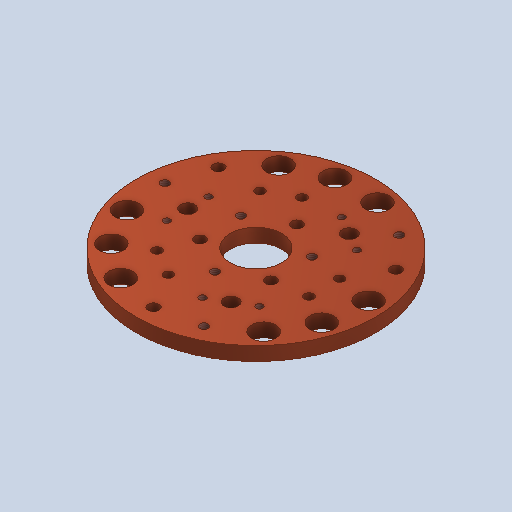
# Autodesk Inventor part: torsosc-frame-plate-v3
Saved by Autodesk Inventor 2026 (Build 300175050, 175E)
## iProperties
Created: 2018-11-20
Part Number: torsosc-frame-plate-v3
Material: Copper
Document SubType Name: Modeling
Designer: schanen
Density: 8.94 g/cm^3
Appearance: Copper - Satin
Mass: 121.653 g
Surface Area: 89.8116 cm^2
Volume: 13.6077 cm^3
Author: schanen
Autodesk Inventor part; units mm, degrees
ref_plane "YZ Plane" through (0, 0, 0) normal (1, 0, 0) x (0, 1, 0)
ref_plane "XZ Plane" through (0, 0, 0) normal (0, 1, 0) x (-1, 0, 0)
ref_plane "XY Plane" through (0, 0, 0) normal (0, 0, 1) x (1, 0, 0)
sketch "Sketch1" plane through (0, 0, 0) normal (0, 1, 0) x (-1, 0, 0)
  circle A0 centre (0, 0) radius 35
  circle A1 centre (0, 0) radius 7.5
  dimension "d0" = 70
  dimension "d129" = 15
  constraints: 2 centre point, 2 coincident
  measures "d0" diameter of A0
  measures "d129" diameter of A1
extrude "Extrusion1" add sketch "Sketch1" along normal blind 4
sketch "Sketch2" plane through (0, 4, 0) normal (0, 1, 0) x (1, 0, 0)
  circle A0 centre (0, 0) radius 30 construction
  point P0 (0, -30)
  point P1 (-25.9808, 15)
  point P2 (25.9808, 15)
  dimension "d130" = 60
  dimension "d131" = 120
  dimension "d132" = 120
  constraints: 3 point on circle, 1 centre point, 1 coincident, 1 vertical alignment
  measures "d130" diameter of A0
hole "Hole1" at (-25.9808, 4, -15) at (25.9808, 4, -15) at (0, 4, 30) direction (0, -1, 0) diameter 3.2 end through all
sketch "Sketch16" plane through (0, 4, 0) normal (0, 1, 0) x (1, 0, 0)
  circle A0 centre (0, 0) radius 12 construction
  point P0 (0, -12)
  point P1 (-10.3923, 6)
  point P2 (10.3923, 6)
  dimension "d155" = 24
  dimension "d156" = 120
  dimension "d157" = 120
  constraints: 3 point on circle, 1 centre point, 1 coincident, 1 vertical alignment
  measures "d155" diameter of A0
hole "Hole14" at (0, 4, 12) at (-10.3923, 4, -6) at (10.3923, 4, -6) direction (0, -1, 0) diameter 2.459 end through all thread size "M3x0.5" class "6H" standard "ISO Metric profile"
sketch "Sketch17" plane through (0, 4, 0) normal (0, 1, 0) x (1, 0, 0)
  circle A0 centre (0, 0) radius 12 construction
  point P0 (0, 12)
  point P1 (-10.3923, -6)
  point P2 (10.3923, -6)
  dimension "d165" = 24
  dimension "d166" = 120
  dimension "d167" = 120
  constraints: 3 point on circle, 1 centre point, 1 coincident, 1 vertical alignment
  measures "d165" diameter of A0
hole "Hole15" at (0, 4, -12) at (-10.3923, 4, 6) at (10.3923, 4, 6) direction (0, -1, 0) diameter 3.2 end through all
sketch "Sketch18" plane through (0, 4, 0) normal (0, 1, 0) x (1, 0, 0)
  point P0 (0, 0)
  point P1 (20, 4.5)
  point P2 (20, -4.5)
  dimension "d175" = 9
  dimension "d176" = 4.5
  dimension "d177" = 20
  measures "d175" distance of point (20, -4.5) point (20, 4.5)
  measures "d176" vertical distance of point (0, 0) point (20, -4.5)
  measures "d177" horizontal distance of point (0, 0) point (20, -4.5)
hole "Hole16" at (20, 4, -4.5) at (20, 4, 4.5) direction (0, -1, 0) diameter 2.7 end through all
sketch "Sketch23" plane through (0, 4, 0) normal (0, 1, 0) x (1, 0, 0)
  point P0 (0, 0)
  point P1 (-20, 0)
  dimension "d238" = 20
  constraints: 1 horizontal alignment
  measures "d238" distance of point (0, 0) point (-20, 0)
hole "Hole21" at (-20, 4, 0) direction (0, -1, 0) diameter 4.2 end through all
sketch "Sketch24" plane through (0, 4, 0) normal (0, 1, 0) x (1, 0, 0)
  circle A0 centre (-20, 0) radius 2.1 projected
  point P0 (0, 0)
  point P1 (-20, 6.1)
  point P2 (-20, -6.1)
  dimension "d246" = 12.2
  dimension "d247" = 6.1
  constraints: 2 vertical alignment
  measures "d246" distance of point (-20, -6.1) point (-20, 6.1)
  measures "d247" distance of A0.centre point (-20, 6.1)
hole "Hole22" at (-20, 4, -6.1) at (-20, 4, 6.1) direction (0, -1, 0) diameter 2.013 end through all thread size "M2.5x0.45" class "6H" standard "ANSI Metric M Profile"
pattern_circular "Circular Pattern6" count 3 over 360 about axis through (0, 0, 0) along (0, 1, 0) of "Hole21", "Hole22"
pattern_circular "Circular Pattern7" count 3 over 360 about axis through (0, 0, 0) along (0, 1, 0) of "Hole16"
sketch "Sketch25" plane through (0, 4, 0) normal (0, 1, 0) x (1, 0, 0)
  circle A0 centre (0, 0) radius 30 construction
  circle A1 centre (0, -30) radius 1.6 projected
  point P0 (12.2021, -27.4064)
  point P1 (22.2943, -20.0739)
  point P2 (28.5317, -9.2705)
  point P3 (29.8357, 3.1359)
  dimension "d261" = 60
  dimension "d262" = 24
  dimension "d263" = 24
  dimension "d264" = 24
  dimension "d275" = 24
  constraints: 4 point on circle, 1 centre point, 1 coincident
  measures "d261" diameter of A0
hole "Hole23" at (22.2943, 4, 20.0739) at (28.5317, 4, 9.2705) at (29.8357, 4, -3.1359) direction (0, -1, 0) diameter 7 end through all
pattern_circular "Circular Pattern8" count 3 over 360 about axis through (0, 0, 0) along (0, 1, 0) of "Hole23"
sketch "Sketch26" plane through (0, 4, 0) normal (0, 1, 0) x (1, 0, 0)
  circle A0 centre (22.2943, -20.0739) radius 3.5 projected
  point P0 (0, 0)
  point P1 (12.2021, -27.4064)
  dimension "d276" = 30
  dimension "d277" = 24
  measures "d276" distance of point (0, 0) point (12.202, -27.406)
hole "Hole24" at (12.2021, 4, 27.4064) direction (0, -1, 0) diameter 2.459 end through all thread size "M3x0.5" class "6H" standard "ISO Metric profile"
pattern_circular "Circular Pattern9" count 3 over 360 about axis through (0, 0, 0) along (0, 1, 0) of "Hole24"
equation "\"d176\" = 0.5 * d175"
equation "\"d247\" = 0.5 * d246"
body "Solid1"
